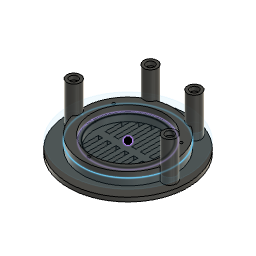
bottom v4 (Autodesk Fusion 360 design; units mm, degrees)
Autodesk Fusion 360 part; units mm, degrees
sketch "Sketch1" plane through (0, 0, 0) normal (0, 0, 1) x (1, 0, 0) in component "corpus"
  circle A0 centre (0, 0) radius 43.5
  line L0 (0, 0) -> (0, 55) construction
  line L1 (0, 43.5) -> (-16, 43.5) construction
  line L2 (-16, 43.5) -> (-16, 0) construction
  line L3 (-16, 40.4506) -> (-16, 32.4506)
  circle A1 centre (-16, 32.4506) radius 5
  circle A2 centre (16, 32.4506) radius 5
  line L4 (-16, 32.4506) -> (16, 32.4506) construction
  line L5 (0, 32.4506) -> (0, -4.5494) construction
  line L6 (0, -4.5494) -> (-35, -4.5494) construction
  circle A3 centre (-35, -4.5494) radius 5
  circle A4 centre (35, -4.5494) radius 5
  dimension "d1" = 87
  dimension "d2" = 16
  dimension "d4" = 8
  dimension "d5" = 10
  dimension "d6" = 37
  dimension "d7" = 35
  dimension "d8" = 10
  constraint coincident A0.centre L0.start
  constraint vertical L0
  constraint coincident A0 L1.start
  constraint coincident L0 L1.start
  constraint perpendicular L0 L1
  constraint perpendicular L1 L2
  constraint coincident L2 L3.start
  constraint coincident A0 L3.start
  constraint parallel L2 L3
  constraint coincident L3.end A1.centre
  constraint symmetric L0 A1 A2
  constraint coincident A2.centre L4.end
  constraint midpoint L4 L5.start
  constraint perpendicular L4 L5
  constraint perpendicular L5 L6
  constraint coincident L6.end A3.centre
  constraint symmetric L5 A3 A4
  measures "d1" diameter of A0
  measures "d2" distance of L1.start L1.end
  measures "d4" distance of L3.start L3.end
  measures "d5" diameter of A1
  measures "d6" distance of L5.start L5.end
  measures "d7" distance of L5.end L6.end
  measures "d8" diameter of A3
extrude "Extrude1" add sketch "Sketch1" against normal blind 3 contours A0 | A1 | A2 | A3 | A4 makes body 1 in component "corpus"
extrude "Extrude2" add sketch "Sketch1" along normal blind 29 contours A1 | A2 | A3 | A4 bodies 1 in component "corpus"
sketch "Sketch2" plane through (0, 0, -3) normal (0, 0, -1) x (1, 0, 0) in component "corpus"
  circle A0 centre (0, 0) radius 43.5
sketch "Sketch3" plane through (0, 0, 0) normal (0, 0, 1) x (1, 0, 0) in component "corpus"
  circle A0 centre (35, -4.5494) radius 3
  circle A1 centre (16, 32.4506) radius 3
  circle A2 centre (-16, 32.4506) radius 3
  circle A3 centre (-35, -4.5494) radius 3
  point P0 (-35, -4.5494)
  point P1 (-16, 32.4506)
  point P2 (16, 32.4506)
  point P3 (35, -4.5494)
  dimension "d13" = 6
  dimension "d14" = 6
  dimension "d15" = 6
  dimension "d16" = 6
  constraint coincident P3 A0.centre
  constraint coincident P2 A1.centre
  constraint coincident P1 A2.centre
  constraint coincident P0 A3.centre
  measures "d13" diameter of A0
  measures "d14" diameter of A1
  measures "d15" diameter of A2
  measures "d16" diameter of A3
extrude "Extrude3" cut sketch "Sketch3" along normal up to surface (23 mm away) and the other way up to surface (3 mm away) bodies 1 in component "corpus"
hole "Hole1" at (16, 32.4506, 0) at (-16, 32.4506, 0) at (-35, -4.5494, 0) at (35, -4.5494, 0) direction (0, 0, 1) diameter 2 depth 30 tip angle 118 bodies 1 in component "corpus"
sketch "Sketch1 (2)" plane through (0, 0, 0) normal (0, 0, 1) x (1, 0, 0) in component "speaker"
  circle A0 centre (0, 0) radius 26
  dimension "d24" = 52
  constraint coincident A0.centre origin
  measures "d24" diameter of A0
extrude "Extrude1'" add sketch "Sketch1 (2)" along normal blind 3 separate body makes body 2 in component "speaker"
ref_plane "WorkPlane1" through (0, 0, 13) normal (0, 0, 1) x (1, 0, 0) in component "speaker"
sketch "Sketch2 (2)" plane through (0, 0, 13) normal (0, 0, 1) x (1, 0, 0) in component "speaker"
  circle A0 centre (0, 0) radius 20
  dimension "d28" = 40
  constraint coincident A0.centre origin
  measures "d28" diameter of A0
extrude "Extrude2'" add sketch "Sketch2 (2)" along normal blind 18 separate body makes body 3 in component "speaker"
loft "Loft1" add section 1 face at (4.3333, 7.5056, 3) section 2 face at (4.7423, -7.1112, 13) separate body on bodies 2 3 makes body 4 in component "speaker"
sketch "Sketch1 (3)" plane through (0, 0, 0) normal (0, 0, 1) x (-1, 0, 0) in component "speaker-holder"
  circle A0 centre (35, 4.5494) radius 5
  circle A1 centre (-35, 4.5494) radius 5
  circle A2 centre (16, -32.4506) radius 5
  circle A3 centre (-16, -32.4506) radius 5
  circle A4 centre (0, 0) radius 43.5
  circle A5 centre (0, 0) radius 33.3166
  circle A6 centre (0, 0) radius 26
  circle A7 centre (0, 0) radius 24
  dimension "d37" = 48
  constraint coincident A4.centre A5.centre
  measures "d37" diameter of A7
extrude "Extrude1''" add sketch "Sketch1 (3)" along normal blind 4 separate body contours A0 A1 A2 A3 A5 makes body 5 in component "speaker-holder"
move_face "OffsetFaces1" offset -0.5 1 faces at (25.8708, 2.5888, 1.3333) on bodies 5 in component "speaker-holder"
sketch "Sketch4" plane through (0, 0, -3) normal (0, 0, -1) x (1, 0, 0) in component "corpus"
  circle A0 centre (-16, -32.4506) radius 3
  circle A1 centre (16, -32.4506) radius 3
  circle A2 centre (-35, 4.5494) radius 3
  circle A3 centre (35, 4.5494) radius 3
  circle A4 centre (0, 0) radius 43.5
  circle A5 centre (0, 0) radius 24
  line L0 (-25.5, 27) -> (-22.5, 27)
  line L1 (-22.5, 27) -> (-22.5, -27)
  line L2 (-22.5, -27) -> (-25.5, -27)
  line L3 (-25.5, -27) -> (-25.5, 27)
  line L4 (-25.5, 27) -> (-22.5, -27) construction
  line L5 (-22.5, 27) -> (-25.5, -27) construction
  line L6 (-16.0714, 27) -> (-16.0714, -27)
  line L7 (-19.0714, 27) -> (-16.0714, 27)
  line L8 (-19.0714, -27) -> (-19.0714, 27)
  line L9 (-16.0714, -27) -> (-19.0714, -27)
  line L10 (-9.6429, 27) -> (-9.6429, -27)
  line L11 (-12.6429, 27) -> (-9.6429, 27)
  line L12 (-12.6429, -27) -> (-12.6429, 27)
  line L13 (-9.6429, -27) -> (-12.6429, -27)
  line L14 (-3.2143, 27) -> (-3.2143, -27)
  line L15 (-6.2143, 27) -> (-3.2143, 27)
  line L16 (-6.2143, -27) -> (-6.2143, 27)
  line L17 (-3.2143, -27) -> (-6.2143, -27)
  line L18 (3.2143, 27) -> (3.2143, -27)
  line L19 (0.2143, 27) -> (3.2143, 27)
  line L20 (0.2143, -27) -> (0.2143, 27)
  line L21 (3.2143, -27) -> (0.2143, -27)
  line L22 (9.6429, 27) -> (9.6429, -27)
  line L23 (6.6429, 27) -> (9.6429, 27)
  line L24 (6.6429, -27) -> (6.6429, 27)
  line L25 (9.6429, -27) -> (6.6429, -27)
  line L26 (16.0714, 27) -> (16.0714, -27)
  line L27 (13.0714, 27) -> (16.0714, 27)
  line L28 (13.0714, -27) -> (13.0714, 27)
  line L29 (16.0714, -27) -> (13.0714, -27)
  line L30 (22.5, 27) -> (22.5, -27)
  line L31 (19.5, 27) -> (22.5, 27)
  line L32 (19.5, -27) -> (19.5, 27)
  line L33 (22.5, -27) -> (19.5, -27)
  line L34 (28.6985, -2.5154) -> (-28.6985, -2.5154)
  line L35 (-28.6985, -2.5154) -> (-28.6985, 2.5154)
  line L36 (-28.6985, 2.5154) -> (28.6985, 2.5154)
  line L37 (28.6985, 2.5154) -> (28.6985, -2.5154)
  line L38 (28.6985, -2.5154) -> (-28.6985, 2.5154) construction
  line L39 (-28.6985, -2.5154) -> (28.6985, 2.5154) construction
  point P0 (-24, 0)
  dimension "d34" = 48
  dimension "d40" = 3
  dimension "d41" = 54
  dimension "d44" = 45
  dimension "d45" = 0
  constraint coincident A4.centre A5.centre
  constraint horizontal L0
  constraint perpendicular L0 L1
  constraint parallel L0 L2
  constraint parallel L1 L3
  constraint coincident L4 P0
  constraint coincident L5 P0
  constraint coincident A5 P0
  constraint horizontal L34
  constraint perpendicular L34 L35
  constraint parallel L34 L36
  constraint parallel L35 L37
  constraint coincident L38 A4.centre
  constraint coincident L39 A4.centre
  measures "d34" diameter of A5
  measures "d40" distance of L1.end L2.end
  measures "d41" distance of L0.end L1.end
extrude "Extrude2''" add 1 faces at (-30.3981, 2.7581, 0) along direction (0, 0, -1) up to surface (5 mm away) on bodies 5 bodies 5 in component "speaker-holder"
extrude "Extrude3'" add sketch "Sketch1 (3)" against normal up to surface (5 mm away) separate body contours A6 makes body 6 in component "speaker-holder"
extrude "Extrude4" cut sketch "Sketch4" against normal blind 13 contours A5 L30 L32 L36 | A5 L30 L32 L34 | A5 L26 L28 L36 | A5 L26 L28 L34 | A5 L22 L24 L36 | A5 L22 L24 L34 | A5 L18 L20 L36 | A5 L18 L20 L34 | A5 L14 L16 L36 | A5 L14 L16 L34 | A5 L10 L12 L36 | A5 L10 L12 L34 | A5 L6 L8 L36 | A5 L6 L8 L34 bodies 1 in component "corpus"
sketch "Sketch1 (4)" plane through (0, 0, 29) normal (0, 0, 1) x (-1, 0, 0)
  circle A0 centre (-35, 4.5494) radius 1
  circle A1 centre (-35, 4.5494) radius 5
  circle A2 centre (-35, 4.5494) radius 3
  circle A3 centre (-16, -32.4506) radius 3
  circle A4 centre (16, -32.4506) radius 3
  circle A5 centre (35, 4.5494) radius 3
  point P0 (-16, -32.4506)
  point P1 (16, -32.4506)
  point P2 (35, 4.5494)
  dimension "d48" = 6
  dimension "d49" = 6
  dimension "d50" = 6
  dimension "d51" = 6
  constraint concentric A0 A2
  constraint coincident P0 A3.centre
  constraint coincident P1 A4.centre
  constraint coincident P2 A5.centre
  measures "d48" diameter of A2
  measures "d49" diameter of A3
  measures "d50" diameter of A4
  measures "d51" diameter of A5
extrude "Extrude5" cut sketch "Sketch1 (4)" against normal blind 3 contours A2 | A3 | A4 | A5 bodies 1 in component "corpus"
sketch "Sketch2 (3)" plane through (0, 0, 4) normal (0, 0, 1) x (-1, 0, 0) in component "speaker-holder"
  circle A0 centre (0, 0) radius 26.5
  arc A1 (-33.3162, -0.1585) -> (-18.152, -27.9374) centre (0, 0) ccw
  arc A2 (-11.1095, -31.4098) -> (-18.152, -27.9374) centre (-16, -32.4506) ccw
  arc A3 (-11.1095, -31.4098) -> (11.1095, -31.4098) centre (0, 0) ccw
  arc A4 (18.152, -27.9374) -> (11.1095, -31.4098) centre (16, -32.4506) ccw
  arc A5 (18.152, -27.9374) -> (33.3162, -0.1585) centre (0, 0) ccw
  arc A6 (32.1686, 8.6705) -> (33.3162, -0.1585) centre (35, 4.5494) ccw
  arc A7 (32.1686, 8.6705) -> (-32.1686, 8.6705) centre (0, 0) ccw
  arc A8 (-33.3162, -0.1585) -> (-32.1686, 8.6705) centre (-35, 4.5494) ccw
  circle A9 centre (0, 0) radius 28.5
  line L0 (0, 0) -> (0, 32) construction
  point P0 (0, 28.5)
  dimension "d54" = 2
  constraint coincident A0.centre A1.centre
  constraint vertical L0
  constraint coincident A9 P0
  constraint coincident L0 P0
hole "Hole1'" at (0, -28.5, 4) direction (0, 0, -1) diameter 2 depth 5 tip angle 118 bodies 5 in component "speaker-holder"
pattern_circular "C-Pattern1" count 3 over 360 about axis through (0, 0, 1.75) along (0, 0, 1) of "Hole1'" in component "speaker-holder"
combine "Combine1" [suppressed] in component "speaker-holder"
component "corpus" placed x (1, 0, 0) y (0, 1, 0) z (0, 0, 1) at (0, 0, 0)
component "speaker" placed x (1, 0, 0) y (0, 1, 0) z (0, 0, 1) at (0, 0, 5)
component "speaker-holder" placed x (1, 0, 0) y (0, 1, 0) z (0, 0, 1) at (0, 0, 5) in component "corpus"
equation "d11 = 32 mm - 3 mm"
